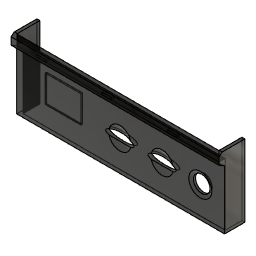
ks-330-io-panel-overlay-1.0-dev (Autodesk Fusion 360 design; units mm, degrees)
Autodesk Fusion 360 part; units mm, degrees
sketch "Front-Base" plane through (0, 0, 0) normal (0, 1, 0) x (1, 0, 0)
  line L0 (-74.9, -0.12) -> (74.9, -0.12)
  line L1 (74.9, -0.12) -> (74.9, -52.12)
  line L2 (74.9, -52.12) -> (-74.9, -52.12)
  line L3 (-74.9, -52.12) -> (-74.9, -0.12)
  dimension "d1" = 149.8
  dimension "d2" = 52
  dimension "d3" = 74.9
  constraint horizontal L0
  constraint vertical L1
  constraint horizontal L2
  constraint vertical L3
  measures "d1" distance of L0.start L0.end
  measures "d2" distance of L0.start L2.end
  measures "d3" distance of origin L1
extrude "Extrude1" add sketch "Front-Base" along normal blind 2.54
sketch "Back-Ears" plane through (0, 2.54, 0) normal (0, 1, 0) x (-1, 0, 0)
  line L0 (74.9, 52.12) -> (-74.9, 52.12)
  line L1 (-74.9, 52.12) -> (-74.9, 0.12)
  line L2 (-74.9, 0.12) -> (74.9, 0.12)
  line L3 (74.9, 0.12) -> (74.9, 52.12)
  line L4 (-74.9, 52.12) -> (-72.78, 52.12)
  line L5 (-72.78, 52.12) -> (-72.78, 0.12)
  line L6 (-72.78, 0.12) -> (-74.9, 0.12)
  line L7 (-74.9, 0.12) -> (-74.9, 52.12)
  line L8 (74.9, 52.12) -> (72.78, 52.12)
  line L9 (72.78, 52.12) -> (72.78, 0.12)
  line L10 (72.78, 0.12) -> (74.9, 0.12)
  line L11 (74.9, 0.12) -> (74.9, 52.12)
  line L12 (74.9, 52.12) -> (-74.9, 52.12)
  line L13 (-74.9, 52.12) -> (-74.9, 45.1516)
  line L14 (-74.9, 45.1516) -> (74.9, 45.1516)
  line L15 (74.9, 45.1516) -> (74.9, 52.12)
  dimension "d7" = 2.12
  dimension "d8" = 2.12
  constraint horizontal L4
  constraint vertical L5
  constraint horizontal L6
  constraint vertical L7
  constraint coincident L0.end L1.start
  constraint horizontal L8
  constraint vertical L9
  constraint horizontal L10
  constraint vertical L11
  constraint coincident L0.start L3.end
  constraint horizontal L12
  constraint vertical L13
  constraint horizontal L14
  constraint vertical L15
  constraint coincident L7 L13.end
  measures "d7" distance of L0.end L4.end
  measures "d8" distance of L0.start L8.end
sketch "LEDSection-Front-Extrusion" plane through (0, 0, 0) normal (0, -1, 0) x (1, 0, 0)
  line L0 (74.9, 52.12) -> (-74.9, 52.12)
  line L1 (-74.9, 52.12) -> (-74.9, 0.12)
  line L2 (-74.9, 0.12) -> (74.9, 0.12)
  line L3 (74.9, 0.12) -> (74.9, 52.12)
  line L4 (-74.9, 52.12) -> (74.9, 52.12)
  line L5 (74.9, 52.12) -> (74.9, 42.62)
  line L6 (74.9, 42.62) -> (-74.9, 42.62)
  line L7 (-74.9, 42.62) -> (-74.9, 52.12)
  dimension "d9" = 9.5
  constraint horizontal L4
  constraint vertical L5
  constraint horizontal L6
  constraint vertical L7
  constraint coincident L0.end L1.start
  measures "d9" distance of L0.end L6.end
extrude "Extrude2" add sketch "LEDSection-Front-Extrusion" along normal blind 4 contours L0 L1 L3 L4 L5 L6 L7
extrude "Extrude3" add sketch "Back-Ears" along normal blind 12.065 contours L0 L3 L8 L9 L11 L12 L14 L15 | L2 L3 L9 L10 L11 L14 | L0 L1 L4 L5 L7 L12 L13 L14 | L1 L2 L5 L6 L7 L14
sketch "LEDSection-Right-Chamfer" plane through (74.9, 0, 0) normal (1, 0, 0) x (0, 1, 0)
  line L0 (0, 42.62) -> (0, 0.12)
  line L1 (0, 0.12) -> (14.605, 0.12)
  line L2 (14.605, 0.12) -> (14.605, 52.12)
  line L3 (14.605, 52.12) -> (-4, 52.12)
  line L4 (-4, 52.12) -> (-4, 42.62)
  line L5 (-4, 42.62) -> (0, 42.62)
  line L6 (0, 42.62) -> (-4, 44.9294)
  line L7 (0, 42.62) -> (4.6188, 42.62) construction
  line L8 (-1.75, 52.12) -> (-4, 50.232)
  line L9 (-1.75, 52.12) -> (-5.2322, 52.12) construction
  line L10 (-4, 52.12) -> (-1.75, 52.12)
  line L11 (-4, 50.232) -> (-4, 52.12)
  line L12 (-4, 44.9294) -> (-4, 42.62)
  line L13 (0, 42.62) -> (-4, 42.62)
  dimension "d14" = 150
  dimension "d15" = 40
  dimension "d16" = 2.25
  constraint horizontal L7
  constraint coincident L0.start L5.end
  constraint coincident L4 L6.end
  constraint horizontal L9
  constraint coincident L3 L8.start
  constraint coincident L4 L8.end
  constraint coincident L3.end L4.start
  constraint coincident L4.end L5.start
  measures "d14" angle of L6 L7
  measures "d15" angle of L8 L9
  measures "d16" horizontal distance of L8.start L8.end
extrude "Extrude4" cut sketch "LEDSection-Right-Chamfer" against normal blind 150 contours L4 L5 L6 L12 L13 | L3 L4 L8 L10 L11
sketch "LEDSection-Back-Lowering" plane through (0, 2.54, 0) normal (0, 1, 0) x (-1, 0, 0)
  line L0 (72.78, 0.12) -> (72.78, 52.12)
  line L1 (72.78, 52.12) -> (-72.78, 52.12)
  line L2 (-72.78, 52.12) -> (-72.78, 0.12)
  line L3 (-72.78, 0.12) -> (72.78, 0.12)
  line L4 (-72.78, 52.12) -> (72.78, 52.12)
  line L5 (72.78, 52.12) -> (72.78, 44.9322)
  line L6 (72.78, 44.9322) -> (-72.78, 44.9322)
  line L7 (-72.78, 44.9322) -> (-72.78, 52.12)
  constraint horizontal L4
  constraint vertical L5
  constraint horizontal L6
  constraint vertical L7
  constraint coincident L0 L5.end
  constraint coincident L1.end L2.start
extrude "Extrude5" cut sketch "LEDSection-Back-Lowering" against normal blind 4.445 contours L0 L1 L2 L4 L5 L6 L7
sketch "LEDSection-Left-InnerChamfer" plane through (-74.9, 0, 0) normal (-1, 0, 0) x (0, -1, 0)
  line L0 (4, 50.232) -> (1.75, 52.12)
  line L1 (1.75, 52.12) -> (-14.605, 52.12)
  line L2 (-14.605, 52.12) -> (-14.605, 0.12)
  line L3 (-14.605, 0.12) -> (0, 0.12)
  line L4 (0, 0.12) -> (0, 42.62)
  line L5 (0, 42.62) -> (4, 44.9294)
  line L6 (4, 44.9294) -> (4, 50.232)
  line L7 (1.9053, 51.9897) -> (1.9034, 51.9897)
  line L8 (1.9034, 45.2797) -> (1.9053, 45.2797)
  line L9 (1.9053, 45.2797) -> (1.9053, 51.9897)
  line L10 (1.9053, 45.2797) -> (-2.5437, 42.7111)
  line L11 (-2.5437, 42.7111) -> (-2.5437, 45.2797)
  line L12 (-2.5437, 45.2797) -> (1.9053, 45.2797)
  line L13 (1.9053, 45.2797) -> (1.9053, 44.93)
  line L14 (1.9053, 44.93) -> (1.2996, 44.93)
  dimension "d23" = 6.71
  constraint horizontal L7
  constraint horizontal L8
  constraint vertical L9
  constraint coincident L0 L7.start
  constraint perpendicular L9 L12
  constraint perpendicular L8 L13
  constraint coincident L10 L14.end
  constraint perpendicular L13 L14
  measures "d23" distance of L7.start L8.end
sketch "LEDSection-Back-Cutout" plane through (0, -1.905, 0) normal (0, 1, 0) x (-1, 0, 0)
  line L0 (72.78, 51.9899) -> (-72.78, 51.9899)
  line L1 (-72.78, 51.9899) -> (-72.78, 44.9322)
  line L2 (-72.78, 44.9322) -> (72.78, 44.9322)
  line L3 (72.78, 44.9322) -> (72.78, 51.9899)
  line L4 (-44.28, 48.2399) -> (-37.28, 48.2399)
  line L5 (-37.28, 48.2399) -> (-37.28, 46.6399)
  line L6 (-37.28, 46.6399) -> (-44.28, 46.6399)
  line L7 (-44.28, 46.6399) -> (-44.28, 48.2399)
  line L8 (2.72, 48.2399) -> (9.72, 48.2399)
  line L9 (9.72, 48.2399) -> (9.72, 46.6399)
  line L10 (9.72, 46.6399) -> (2.72, 46.6399)
  line L11 (2.72, 46.6399) -> (2.72, 48.2399)
  line L12 (49.72, 48.2399) -> (56.72, 48.2399)
  line L13 (56.72, 48.2399) -> (56.72, 46.6399)
  line L14 (56.72, 46.6399) -> (49.72, 46.6399)
  line L15 (49.72, 46.6399) -> (49.72, 48.2399)
  dimension "d30" = 7
  dimension "d31" = 1.6
  dimension "d32" = 28.5
  dimension "d33" = 7
  dimension "d34" = 1.6
  dimension "d35" = 40
  dimension "d36" = 7
  dimension "d37" = 1.6
  dimension "d38" = 40
  dimension "d39" = 3.75
  dimension "d40" = 3.75
  dimension "d41" = 3.75
  constraint horizontal L4
  constraint vertical L5
  constraint horizontal L6
  constraint vertical L7
  constraint horizontal L8
  constraint vertical L9
  constraint horizontal L10
  constraint vertical L11
  constraint horizontal L12
  constraint vertical L13
  constraint horizontal L14
  constraint vertical L15
  measures "d30" distance of L4.start L4.end
  measures "d31" distance of L4.start L6.end
  measures "d32" distance of L1 L7
  measures "d33" distance of L8.start L8.end
  measures "d34" distance of L8.start L10.end
  measures "d35" distance of L5 L11
  measures "d36" distance of L12.start L12.end
  measures "d37" distance of L12.start L14.end
  measures "d38" distance of L9 L14.end
  measures "d39" distance of L0 L8
  measures "d40" distance of L0 L4
  measures "d41" distance of L0 L12
extrude "Extrude9" cut sketch "LEDSection-Back-Cutout" against normal blind 1.8 contours L4 L5 L6 L7 | L8 L9 L10 L11 | L12 L13 L14 L15
sketch "IOSection-Back" plane through (0, 2.54, 0) normal (0, 1, 0) x (-1, 0, 0)
  line L0 (72.78, 44.9322) -> (-72.78, 44.9322)
  line L1 (-72.78, 44.9322) -> (-72.78, 0.12)
  line L2 (-72.78, 0.12) -> (72.78, 0.12)
  line L3 (72.78, 0.12) -> (72.78, 44.9322)
  line L4 (30.1, 34.37) -> (55.9, 34.37)
  line L5 (55.9, 34.37) -> (55.9, 14.77)
  line L6 (55.9, 14.77) -> (30.1, 14.77)
  line L7 (30.1, 14.77) -> (30.1, 34.37)
  line L8 (74.9, 0.12) -> (74.9, 52.12)
  line L9 (-57.4, 22.12) -> (14.6, 22.12)
  line L10 (-74.9, 52.12) -> (-74.9, 0.12)
  circle A0 centre (-57.4, 22.12) radius 6
  line L11 (-51.4, 22.12) -> (-40.05, 22.12)
  line L12 (-40.05, 22.12) -> (-19.65, 22.12)
  line L13 (-19.65, 22.12) -> (-19.65, 19.195)
  line L14 (-19.65, 19.195) -> (-40.05, 19.195)
  line L15 (-40.05, 19.195) -> (-40.05, 22.12)
  line L16 (-19.65, 22.12) -> (-9.65, 22.12)
  line L17 (-9.65, 22.12) -> (10.75, 22.12)
  line L18 (10.75, 22.12) -> (10.75, 19.195)
  line L19 (10.75, 19.195) -> (-9.65, 19.195)
  line L20 (-9.65, 19.195) -> (-9.65, 22.12)
  ellipse E0 centre (-29.85, 22.12) end of major axis (-19.65, 22.12) minor radius 2.925
  line L21 (-40.05, 22.12) -> (-19.65, 22.12)
  line L22 (-29.85, 19.195) -> (-29.85, 25.045)
  ellipse E1 centre (0.55, 22.12) end of major axis (10.75, 22.12) minor radius 2.925
  line L23 (-9.65, 22.12) -> (10.75, 22.12)
  line L24 (0.55, 19.195) -> (0.55, 25.045)
  dimension "d44" = 25.8
  dimension "d45" = 19.6
  dimension "d46" = 19
  dimension "d47" = 14.65
  dimension "d50" = 22
  dimension "d51" = 17.5
  dimension "d52" = 12
  dimension "d53" = 11.35
  dimension "d54" = 20.4
  dimension "d55" = 10
  dimension "d56" = 20.4
  dimension "d57" = 2.925
  dimension "d58" = 2.925
  constraint horizontal L4
  constraint vertical L5
  constraint horizontal L6
  constraint vertical L7
  constraint parallel L2 L9
  constraint coincident L9.start A0.centre
  constraint coincident A0 L11.start
  constraint coincident L9 L11.start
  constraint parallel L9 L11
  constraint horizontal L12
  constraint vertical L13
  constraint horizontal L14
  constraint vertical L15
  constraint perpendicular L13 L16
  constraint horizontal L17
  constraint vertical L18
  constraint horizontal L19
  constraint vertical L20
  constraint midpoint L12 E0.centre
  constraint coincident L11.end E0
  constraint coincident L12.end E0
  constraint midpoint L17 E1.centre
  constraint coincident L16.end E1
  constraint coincident E1 L24.start
  constraint coincident E1 L24.end
  measures "d44" distance of L4.start L4.end
  measures "d45" distance of L4.start L6.end
  measures "d46" distance of L5 L8
  measures "d47" distance of L2 L6
  measures "d50" distance of L2 L9
  measures "d51" distance of L9.start L10
  measures "d52" diameter of A0
  measures "d53" distance of L11.start L11.end
  measures "d54" distance of L11.end L12.end
  measures "d55" distance of L12.end L16.end
  measures "d56" distance of L16.end L17.end
  measures "d57" distance of L12 L14
  measures "d58" distance of L17 L19
extrude "Extrude10" cut sketch "IOSection-Back" against normal blind 1 contours L4 L5 L6 L7
extrude "Extrude11" cut sketch "IOSection-Back" against normal blind 2.54 contours L9 L12 E0 L21 L22 | L9 L12 E0 L21 L22 | L9 L12 E0 L21 L22 | L9 L12 E0 L21 L22 | L9 L17 E1 L23 L24 | L9 L17 E1 L23 L24 | L9 L17 E1 L23 L24 | L9 L17 E1 L23 L24 | A0
sketch "IOSection-Front-Detailing" plane through (0, 0, 0) normal (0, -1, 0) x (1, 0, 0)
  ellipse E0 centre (29.85, 22.12) end of major axis (19.65, 22.12) minor radius 2.925
  ellipse E1 centre (-0.55, 22.12) end of major axis (-10.75, 22.12) minor radius 2.925
  circle A0 centre (57.4, 22.12) radius 6
  line L0 (74.9, 42.62) -> (-74.9, 42.62)
  line L1 (-74.9, 42.62) -> (-74.9, 0.12)
  line L2 (-74.9, 0.12) -> (74.9, 0.12)
  line L3 (74.9, 0.12) -> (74.9, 42.62)
  circle A1 centre (-0.55, 22.12) radius 8
  circle A2 centre (29.85, 22.12) radius 8
  dimension "d61" = 16
  dimension "d62" = 16
  constraint concentric E1 A1
  constraint concentric E0 A2
  measures "d61" diameter of A1
  measures "d62" diameter of A2
chamfer "Chamfer2" distance 2.3 distance2 1 1 edges at (62.994, 0, 19.9503) measured on face at (-53.5167, 0, 21.62)
extrude "Extrude12" cut sketch "IOSection-Front-Detailing" against normal blind 1 contours E0 A2 | E0 A2 | E1 A1 | E1 A1 picked at (28.2628, 17.6671) picked at (31.4372, 26.5729) picked at (-2.1372, 17.6671) picked at (1.0372, 26.5729)
fillet "Fillet1" radius 13.33 4 edges at (-0.55, 1, 30.12) (-0.55, 1, 14.12) (29.85, 1, 30.12) (29.85, 1, 14.12)
extrude "Extrude6" [rolled back] along distance -147.7 taper angle 0
extrude "Extrude7" [rolled back] along distance -147.68 taper angle 0
extrude "Extrude8" [rolled back] along distance -2.12 taper angle 0
chamfer "Chamfer1" [rolled back] left distance 2.4 right distance 4.4
equation "d14 = 180 deg - 30 deg"
equation "d51 = 11.5 mm + 6 mm"
equation "d57 = ( 5.85 / 2 ) * 1 mm"
equation "d58 = ( 5.85 / 2 ) * 1 mm"
named bodies: "KS-330-IOPanel-Overlay"
